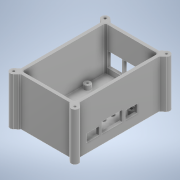
# Autodesk Inventor part: Case RevC
Saved by Autodesk Inventor 2021 (Build 250183000, 183)
## iProperties
Created: 2021-07-24
Part Number: Case RevC
Material: ABS Plastic
Document SubType Name: Modeling
Designer: cmzgt
Density: 0.1 g/cm^3
Appearance: Smooth - White
Author: cmzgt
Autodesk Inventor part; units mm, degrees
ref_plane "YZ Plane" through (0, 0, 0) normal (1, 0, 0) x (0, 1, 0)
ref_plane "XZ Plane" through (0, 0, 0) normal (0, 1, 0) x (-1, 0, 0)
ref_plane "XY Plane" through (0, 0, 0) normal (0, 0, 1) x (1, 0, 0)
sketch "Sketch1" plane through (0, 0, 0) normal (0, 1, 0) x (-1, 0, 0)
  line L0 (-32.55, -49.55) -> (32.55, -49.55)
  line L1 (32.55, -49.55) -> (32.55, 49.55)
  line L2 (32.55, 49.55) -> (-32.55, 49.55)
  line L3 (-32.55, 49.55) -> (-32.55, -49.55)
  line L4 (-32.55, -49.55) -> (32.55, 49.55) construction
  line L5 (32.55, -49.55) -> (-32.55, 49.55) construction
  point P0 (0, 0)
  dimension "d0" = 65.1
  dimension "d1" = 99.1
  constraints: 12 end point, 2 midpoint, 2 parallel, 1 horizontal, 1 perpendicular
  measures "d0" distance of L2.end L1.end
  measures "d1" distance of L0.end L1.end
extrude "Extrusion1" add sketch "Sketch1" along normal blind 5.08
sketch "Sketch2" plane through (0, 5.08, 0) normal (0, 1, 0) x (1, 0, 0)
  line L0 (29.35, 46.35) -> (-29.35, 46.35)
  line L1 (-29.35, 46.35) -> (-29.35, -46.35)
  line L2 (-29.35, -46.35) -> (29.35, -46.35)
  line L3 (29.35, -46.35) -> (29.35, 46.35)
  line L4 (29.35, 46.35) -> (-29.35, -46.35) construction
  line L5 (-29.35, 46.35) -> (29.35, -46.35) construction
  line L6 (-32.55, 49.55) -> (-32.55, -49.55) projected
  line L7 (-32.55, -49.55) -> (32.55, -49.55) projected
  line L8 (32.55, 49.55) -> (-32.55, 49.55) projected
  line L9 (32.55, -49.55) -> (32.55, 49.55) projected
  line L10 (26.15, -43.15) -> (32.55, -49.55) construction
  line L11 (23.6931, -46.35) -> (29.7216, -52.3784)
  line L12 (35.3784, -46.7216) -> (29.35, -40.6931)
  arc A0 (29.7216, -52.3784) -> (35.3784, -46.7216) centre (32.55, -49.55) ccw
  circle A1 centre (32.55, -49.55) radius 1.375
  point P0 (0, 0)
  dimension "d4" = 3.2
  dimension "d5" = 3.2
  dimension "d22" = 8
  dimension "d23" = 2.75
  constraints: 20 end point, 4 parallel, 3 midpoint, 2 centre point, 2 point on circle, 2 point on line, 2 tangent, 1 coincident, 1 horizontal, 1 perpendicular
  measures "d4" distance between parallel lines of L6 L1
  measures "d5" distance between parallel lines of L7 L2
  measures "d22" diameter of A0
  measures "d23" diameter of A1
extrude "Extrusion2" add sketch "Sketch2" along normal blind 48 contours L0 L1 L2 L11 L7 L6 L8 L9 L12 L3 | L12 L9 A1 L7 L11 L2 L3 | L9 L7 A1 picked at (32.448, -48.6448)
sketch "Sketch3" plane through (0, 5.08, 0) normal (0, 1, 0) x (1, 0, 0)
  line L0 (29.35, -46.35) -> (-29.35, -46.35) construction
  line L1 (0, -46.35) -> (0, 46.35) construction
  line L2 (29.35, 46.35) -> (-29.35, 46.35) construction
  circle A0 centre (-24.5, -36.35) radius 3.5
  circle A1 centre (-24.5, -36.35) radius 1.375
  line L3 (29.35, 46.35) -> (29.35, -46.35) construction
  line L4 (29.35, 0) -> (-29.35, 0) construction
  line L5 (-29.35, -46.35) -> (-29.35, 46.35) construction
  circle A2 centre (-24.5, 21.65) radius 3.5
  circle A3 centre (-24.5, 21.65) radius 1.375
  circle A4 centre (24.5, -36.35) radius 3.5
  circle A5 centre (24.5, -36.35) radius 1.375
  circle A6 centre (24.5, 21.65) radius 3.5
  circle A7 centre (24.5, 21.65) radius 1.375
  point P0 (0, 0)
  dimension "d8" = 7
  dimension "d9" = 2.75
  dimension "d10" = 10
  dimension "d11" = 24.5
  dimension "d14" = 58
  constraints: 8 centre point, 4 coincident, 4 end point, 4 midpoint, 4 symmetric about line, 1 vertical, 8 other
  measures "d8" diameter of A0
  measures "d9" diameter of A1
  measures "d10" distance from line of L0 A0.centre
  measures "d11" distance from line of L1 A1.centre
  measures "d14" distance of A0.centre A2.centre
extrude "Extrusion3" add sketch "Sketch3" along normal blind 5
sketch "Sketch4" plane through (0, 0, 0) normal (0, -1, 0) x (1, 0, 0)
  line L0 (31.0438, 48.2342) -> (34.0562, 50.8658) construction
  line L1 (32.55, 49.55) -> (32.55, -49.55) projected
  line L2 (32.55, 44.2386) -> (36.6878, 47.8534)
  line L3 (31.4245, 53.8782) -> (28.4122, 51.2466)
  arc A0 (28.4122, 51.2466) -> (27.2664, 49.55) centre (31.0438, 48.2342) ccw
  arc A1 (36.6878, 47.8534) -> (31.4245, 53.8782) centre (34.0562, 50.8658) ccw
  line L4 (-32.55, 49.55) -> (32.55, 49.55) projected
  line L5 (27.2664, 49.55) -> (32.55, 49.55)
  line L6 (32.55, 49.55) -> (32.55, 44.2386)
  circle A2 centre (34.0562, 50.8658) radius 1.375
  line L7 (0, 49.55) -> (0, -49.55) construction
  line L8 (32.55, -49.55) -> (-32.55, -49.55) construction
  line L9 (32.55, 0) -> (-33.3, 0) construction
  line L10 (32.55, -49.55) -> (32.55, 49.55)
  line L11 (32.55, -44.2386) -> (36.6878, -47.8534)
  line L12 (31.4245, -53.8782) -> (28.4122, -51.2466)
  arc A3 (27.2664, -49.55) -> (28.4122, -51.2466) centre (31.0438, -48.2342) ccw
  arc A4 (31.4245, -53.8782) -> (36.6878, -47.8534) centre (34.0562, -50.8658) ccw
  line L13 (-32.55, -49.55) -> (32.55, -49.55)
  circle A5 centre (34.0562, -50.8658) radius 1.375
  line L14 (-32.55, 49.55) -> (-32.55, -49.55)
  line L15 (-32.55, 44.2386) -> (-36.6878, 47.8534)
  line L16 (-31.4245, 53.8782) -> (-28.4122, 51.2466)
  arc A6 (-27.2664, 49.55) -> (-28.4122, 51.2466) centre (-31.0438, 48.2342) ccw
  arc A7 (-31.4245, 53.8782) -> (-36.6878, 47.8534) centre (-34.0562, 50.8658) ccw
  line L17 (-27.2664, 49.55) -> (-32.55, 49.55)
  circle A8 centre (-34.0562, 50.8658) radius 1.375
  arc A9 (-36.6878, -47.8534) -> (-31.4245, -53.8782) centre (-34.0562, -50.8658) ccw
  line L18 (-32.55, -44.2386) -> (-36.6878, -47.8534)
  line L19 (-31.4245, -53.8782) -> (-28.4122, -51.2466)
  arc A10 (-28.4122, -51.2466) -> (-27.2664, -49.55) centre (-31.0438, -48.2342) ccw
  circle A11 centre (-34.0562, -50.8658) radius 1.375
  line L20 (-27.2664, -49.55) -> (-32.55, -49.55)
  line L21 (-32.55, -49.55) -> (-32.55, 49.55)
  point P0 (0, 0)
  point P1 (-32.55, -44.2386)
  point P2 (-27.2664, 49.55)
  point P3 (32.55, -49.55)
  dimension "d24" = 2
  dimension "d25" = 8
  dimension "d26" = 131.141
  dimension "d27" = 2.75
  constraints: 40 end point, 30 symmetric about line, 16 point on circle, 12 centre point, 6 point on line, 4 coincident, 4 midpoint, 4 tangent, 1 collinear, 1 horizontal, 1 parallel, 9 other
  measures "d24" distance of L1.start L0.end
  measures "d25" diameter of A1
  measures "d26" angle of L1 L2
  measures "d27" diameter of A2
extrude "Extrusion4" add sketch "Sketch4" against normal up to surface (53.08 mm away) contours L4 A0 L3 A1 L2 L1 | L11 A4 L12 A3 L13 L1 | L4 L14 L15 A7 L16 A6 | A10 L19 A9 L18 L14 L13
fillet "Fillet2" radius 2 4 edges at (29.35, 29.08, -46.35) (-29.35, 29.08, -46.35) (-29.35, 29.08, 46.35) (29.35, 29.08, 46.35)
sketch "Sketch5" plane through (0, 5.08, 0) normal (0, 1, 0) x (1, 0, 0)
  line L0 (15, 0) -> (-15, 0) construction
  line L1 (15, 2.5) -> (-15, 2.5)
  line L2 (-15, -2.5) -> (15, -2.5)
  arc A0 (15, -2.5) -> (15, 2.5) centre (15, 0) ccw
  arc A1 (-15, 2.5) -> (-15, -2.5) centre (-15, 0) ccw
  line L3 (-27.35, -46.35) -> (27.35, -46.35) construction
  line L4 (0, -46.35) -> (0, 46.35) construction
  line L5 (-27.35, 46.35) -> (27.35, 46.35) construction
  arc A2 (-15, 12.5) -> (-15, 7.5) centre (-15, 10) ccw
  line L6 (15, 12.5) -> (-15, 12.5)
  line L7 (-15, 7.5) -> (15, 7.5)
  arc A3 (15, 7.5) -> (15, 12.5) centre (15, 10) ccw
  arc A4 (-15, 22.5) -> (-15, 17.5) centre (-15, 20) ccw
  line L8 (15, 22.5) -> (-15, 22.5)
  line L9 (-15, 17.5) -> (15, 17.5)
  arc A5 (15, 17.5) -> (15, 22.5) centre (15, 20) ccw
  arc A6 (-15, 32.5) -> (-15, 27.5) centre (-15, 30) ccw
  line L10 (15, 32.5) -> (-15, 32.5)
  line L11 (-15, 27.5) -> (15, 27.5)
  arc A7 (15, 27.5) -> (15, 32.5) centre (15, 30) ccw
  arc A8 (-15, -7.5) -> (-15, -12.5) centre (-15, -10) ccw
  line L12 (-15, -12.5) -> (15, -12.5)
  line L13 (15, -7.5) -> (-15, -7.5)
  arc A9 (15, -12.5) -> (15, -7.5) centre (15, -10) ccw
  arc A10 (-15, -17.5) -> (-15, -22.5) centre (-15, -20) ccw
  line L14 (-15, -22.5) -> (15, -22.5)
  line L15 (15, -17.5) -> (-15, -17.5)
  arc A11 (15, -22.5) -> (15, -17.5) centre (15, -20) ccw
  arc A12 (-15, -27.5) -> (-15, -32.5) centre (-15, -30) ccw
  line L16 (-15, -32.5) -> (15, -32.5)
  line L17 (15, -27.5) -> (-15, -27.5)
  arc A13 (15, -32.5) -> (15, -27.5) centre (15, -30) ccw
  point P0 (0, 0)
  dimension "d31" = 15
  dimension "d32" = 5
  dimension "d35" = 10
  dimension "d42" = 10
  constraints: 34 end point, 28 point on circle, 14 centre point, 4 tangent, 3 midpoint, 2 vertical, 1 horizontal, 1 parallel, 60 other
  measures "d31" distance of point (0, 0) L0.end
  measures "d32" diameter of A1
  measures "d35" distance of L0.end A2.centre
  measures "d42" distance of L0.end A8.centre
extrude "Extrusion5" cut sketch "Sketch5" against normal up to surface (5.08 mm away)
sketch "Sketch9" plane through (27.2664, 0, -49.55) normal (0, 0, -1) x (-1, 0, 0)
  line L0 (6.2664, 10.08) -> (-0.7336, 10.08) projected
  line L1 (1.3914, 10.08) -> (4.1414, 10.08) projected
  line L2 (1.3914, 10.08) -> (4.1414, 10.08) construction
  line L3 (2.7664, 10.08) -> (-0.7336, 10.08) construction
  line L4 (6.2664, 10.08) -> (-0.7336, 10.08) projected
  line L5 (0, 53.08) -> (0, 0) projected
  line L6 (-0.7336, 10.08) -> (0, 13.5023) construction
  line L7 (17.325, 11.35) -> (1.075, 11.35)
  line L8 (1.075, 11.35) -> (1.075, 25.6)
  line L9 (1.075, 25.6) -> (17.325, 25.6)
  line L10 (17.325, 25.6) -> (17.325, 11.35)
  line L11 (9.2, 25.6) -> (9.2, 11.35) construction
  line L12 (19.875, 11.35) -> (36.125, 11.35)
  line L13 (36.125, 11.35) -> (36.125, 27.85)
  line L14 (36.125, 27.85) -> (19.875, 27.85)
  line L15 (19.875, 27.85) -> (19.875, 11.35)
  line L16 (28, 27.85) -> (28, 11.35) construction
  line L17 (54.125, 27.85) -> (37.875, 27.85)
  line L18 (54.125, 11.35) -> (54.125, 27.85)
  line L19 (37.875, 11.35) -> (54.125, 11.35)
  line L20 (37.875, 27.85) -> (37.875, 11.35)
  point P0 (27.2664, 0)
  point P1 (46, 27.85)
  point P2 (46, 11.35)
  dimension "d58" = 3.5
  dimension "d60" = 3.5
  dimension "d63" = 16.25
  dimension "d64" = 14.25
  dimension "d65" = 1.27
  dimension "d66" = 9.2
  dimension "d69" = 16.25
  dimension "d70" = 16.5
  dimension "d71" = 1.27
  dimension "d72" = 28
  dimension "d75" = 18
  constraints: 32 end point, 5 midpoint, 4 parallel, 3 horizontal, 2 perpendicular, 1 collinear, 1 point on line, 10 other
  measures "d58" distance of L3.start L0.end
  measures "d60" distance of L0.end L6.end
  measures "d63" distance of L8.end L9.end
  measures "d64" distance of L7.end L8.end
  measures "d65" distance between parallel lines of L0 L7
  measures "d66" distance between parallel lines of L5 L11
  measures "d69" distance of L14.end L13.end
  measures "d70" distance of L12.end L13.end
  measures "d71" distance between parallel lines of L4 L12
  measures "d72" distance between parallel lines of L5 L16
  measures "d75" distance of L13.end L17.start
extrude "Extrusion7" cut sketch "Sketch9" against normal up to surface (3.2 mm away)
sketch "Sketch12" plane through (32.55, 0, 44.2386) normal (1, 0, 0) x (0, 0, -1)
  line L0 (0, 53.08) -> (0, 0) projected
  line L1 (28.8305, 16.69) -> (28.8305, 14.2116) projected
  line L2 (43.8305, 14.2116) -> (43.8305, 16.69) projected
  line L3 (10.9402, 12.8971) -> (10.9402, 13.09) projected
  line L4 (18.9209, 13.09) -> (18.9209, 12.8971) projected
  line L5 (54.4305, 17.41) -> (54.4305, 11.41) projected
  line L6 (61.4305, 11.41) -> (61.4305, 17.41) projected
  line L7 (11.9305, 14.1354) -> (17.9305, 14.1354) projected
  line L8 (21.7386, 5.08) -> (26.7386, 5.08) projected
  line L9 (26.7386, 5.08) -> (21.7386, 5.08) projected
  line L10 (41.7386, 5.08) -> (46.7386, 5.08) projected
  line L11 (46.7386, 5.08) -> (41.7386, 5.08) projected
  line L12 (51.7386, 5.08) -> (56.7386, 5.08) projected
  line L13 (56.7386, 5.08) -> (51.7386, 5.08) projected
  line L14 (61.7386, 5.08) -> (66.7386, 5.08) projected
  line L15 (66.7386, 5.08) -> (61.7386, 5.08) projected
  line L16 (11.7386, 5.08) -> (16.7386, 5.08) projected
  line L17 (16.7386, 5.08) -> (11.7386, 5.08) projected
  line L18 (31.7386, 5.08) -> (36.7386, 5.08) projected
  line L19 (36.7386, 5.08) -> (31.7386, 5.08) projected
  line L20 (71.7386, 5.08) -> (76.7386, 5.08) projected
  line L21 (76.7386, 5.08) -> (71.7386, 5.08) projected
  line L22 (4.3886, 5.08) -> (11.3886, 5.08) projected
  line L23 (4.3886, 5.08) -> (11.3886, 5.08) projected
  line L24 (62.3886, 5.08) -> (69.3886, 5.08) projected
  line L25 (62.3886, 5.08) -> (69.3886, 5.08) projected
  line L26 (-2.1114, 5.08) -> (-0.1114, 5.08) projected
  line L27 (-0.1114, 5.08) -> (88.5886, 5.08) projected
  line L28 (88.5886, 5.08) -> (90.5886, 5.08) projected
  line L29 (90.5886, 5.08) -> (88.5886, 5.08) projected
  line L30 (88.5886, 5.08) -> (-0.1114, 5.08) projected
  line L31 (-0.1114, 5.08) -> (-2.1114, 5.08) projected
  line L32 (6.5136, 10.08) -> (9.2636, 10.08) projected
  line L33 (10.9402, 12.9936) -> (18.9209, 12.9936) construction
  line L34 (14.9305, 14.1354) -> (14.9305, 12.9936) construction
  line L35 (7.9402, 19.08) -> (21.9209, 19.08)
  line L36 (21.9209, 19.08) -> (21.9209, 10.08)
  line L37 (21.9209, 10.08) -> (7.9402, 10.08)
  line L38 (7.9402, 10.08) -> (7.9402, 19.08)
  line L39 (43.0305, 17.49) -> (29.6305, 17.49) projected
  line L40 (47.8305, 10.08) -> (24.8305, 10.08)
  line L41 (24.8305, 10.08) -> (24.8305, 22.08)
  line L42 (24.8305, 22.08) -> (47.8305, 22.08)
  line L43 (47.8305, 22.08) -> (47.8305, 10.08)
  line L44 (61.4305, 17.41) -> (57.9305, 17.41) projected
  line L45 (64.4305, 10.08) -> (51.4305, 10.08)
  line L46 (51.4305, 10.08) -> (51.4305, 19.68)
  line L47 (51.4305, 19.68) -> (64.4305, 19.68)
  line L48 (64.4305, 19.68) -> (64.4305, 10.08)
  point P0 (44.2386, 0)
  dimension "d99" = 3
  dimension "d100" = 3
  dimension "d101" = 0
  dimension "d102" = 9
  dimension "d103" = 4
  dimension "d104" = 4
  dimension "d105" = 0
  dimension "d106" = 12
  dimension "d108" = 3
  dimension "d109" = 3
  dimension "d110" = 0
  dimension "d111" = 9.6
  constraints: 28 end point, 6 parallel, 4 midpoint, 3 horizontal, 3 perpendicular
  measures "d99" distance from line of L4.end L36
  measures "d100" distance between parallel lines of L38 L3
  measures "d101" distance between parallel lines of L32 L37
  measures "d102" distance of L37.end L35.start
  measures "d103" distance between parallel lines of L43 L2
  measures "d104" distance between parallel lines of L41 L1
  measures "d105" distance between parallel lines of L32 L40
  measures "d106" distance of L40.end L41.end
  measures "d108" distance between parallel lines of L48 L6
  measures "d109" distance between parallel lines of L5 L46
  measures "d110" distance between parallel lines of L32 L45
  measures "d111" distance of L45.end L46.end
extrude "Extrusion9" cut sketch "Sketch12" against normal up to surface (3.2 mm away)
body "Solid1"
